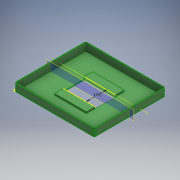
# Autodesk Inventor part: couvercle
Saved by Autodesk Inventor 2017 (Build 210142000, 142)
## iProperties
Part Number: couvercle
Material: Plastique ABS
Document SubType Name: Modeling
Designer: starl
Density: 1.06 g/cm^3
Appearance: Lisse - Blanc
Author: starl
Autodesk Inventor part; units mm, degrees
ref_plane "YZ Plane" through (0, 0, 0) normal (1, 0, 0) x (0, 1, 0)
ref_plane "XZ Plane" through (0, 0, 0) normal (0, 1, 0) x (-1, 0, 0)
ref_plane "XY Plane" through (0, 0, 0) normal (0, 0, 1) x (1, 0, 0)
sketch "Esquisse1" plane through (0, 0, 0) normal (0, 0, 1) x (1, 0, 0)
  line L0 (0, 0) -> (93, 0)
  line L1 (93, 0) -> (93, 83)
  line L2 (93, 83) -> (0, 83)
  line L3 (0, 83) -> (0, 0)
  line L4 (1, 1) -> (92, 1)
  line L5 (92, 1) -> (92, 82)
  line L6 (92, 82) -> (1, 82)
  line L7 (1, 82) -> (1, 1)
  dimension "d0" = 93
  dimension "d1" = 91
  dimension "d2" = 83
  dimension "d3" = 81
  dimension "d4" = 1
  dimension "d5" = 1
  constraints: 16 end point, 4 parallel, 2 horizontal, 2 perpendicular
  measures "d0" distance of L0.start L0.end
  measures "d1" distance of L4.start L4.end
  measures "d2" distance of L0.end L1.end
  measures "d3" distance of L4.end L5.end
  measures "d4" distance between parallel lines of L2 L6
  measures "d5" distance between parallel lines of L3 L7
extrude "Extrusion1" add sketch "Esquisse1" along normal blind 10 contours L3 L2 L1 L0 | L7 L6 L5 L4
shell "Coque1" thickness 1 removed faces 1 at (31, 55.3333, 10)
sketch "Esquisse2" plane through (1, 1, 1) normal (0, 0, 1) x (1, 0, 0)
  point P0 (-1, -1)
sketch "Esquisse3" plane through (1, 1, 1) normal (0, 0, 1) x (1, 0, 0)
  line L0 (63.2856, 52.5) -> (26.2856, 52.5)
  line L1 (26.2856, 52.5) -> (26.2856, 62.5)
  line L2 (26.2856, 62.5) -> (63.2856, 62.5)
  line L3 (63.2856, 62.5) -> (63.2856, 52.5)
  line L4 (0, 0) -> (91, 0) projected
  line L5 (91, 81) -> (0, 81) projected
  line L6 (0, 81) -> (0, 0) projected
  line L7 (92, -1) -> (92, 82) projected
  point P0 (-1, -1)
  point P1 (45.5, 0)
  point P2 (44.7856, 21.5)
  point P3 (44.7856, 52.5)
  point P4 (45.5, 81)
  point P5 (0, 40.5)
  point P6 (92, 40.5)
  point P7 (26.2856, 57.5)
  point P8 (-34.8368, 34.987)
  dimension "d11" = 37
  dimension "d12" = 10
  constraints: 8 end point, 6 midpoint, 2 parallel, 1 horizontal, 1 perpendicular
  measures "d11" distance of L0.start L0.end
  measures "d12" distance of L0.end L1.end
sketch "Esquisse4" plane through (1, 1, 1) normal (0, 0, 1) x (1, 0, 0)
  point P0 (-1, -1)
extrude "Extrusion3" add sketch "Esquisse3" along normal blind 2
shell "Coque3" thickness 0.2 removed faces 1 at (51.9523, 53.5, 1.6667)
ref_plane "Plan de construction1" through (1, 41.5, 1) normal (0, 1, 0) x (1, 0, 0)
mirror "Symétrie1" about plane through (1, 41.5, 1) normal (0, 1, 0) of "Extrusion3"
shell "Coque4" thickness 0.2 removed faces 1 at (51.9523, 29.5, 1.6667)
sketch "Esquisse5" plane through (1, 1, 3) normal (0, 0, 1) x (1, 0, 0)
  line L0 (26.2856, 52.5) -> (63.2856, 52.5) projected
  line L1 (26.2856, 28.5) -> (63.2856, 28.5) projected
  point P0 (-1, -1)
  dimension "d22" = 24
  measures "d22" distance between parallel lines of L0 L1
sketch "Esquisse6" plane through (0, 0, 0) normal (0, 0, -1) x (-1, 0, 0)
  line L0 (-64.2856, 53.5) -> (-28.2856, 53.5)
  line L1 (-28.2856, 53.5) -> (-28.2856, 29.5)
  line L2 (-28.2856, 29.5) -> (-64.2856, 29.5)
  line L3 (-64.2856, 29.5) -> (-64.2856, 53.5)
  line L4 (-64.0856, 53.5) -> (-27.4856, 53.5) projected
  line L5 (-64.2856, 29.5) -> (-64.2856, 19.5) projected
  point P0 (0, 0)
  dimension "d23" = 36
  dimension "d24" = 24
  constraints: 8 end point, 2 collinear, 2 parallel, 1 horizontal, 1 perpendicular
  measures "d23" distance of L0.start L0.end
  measures "d24" distance of L0.end L1.end
extrude "Extrusion4" cut sketch "Esquisse6" against normal blind 2
fillet "Congé1" radius 2 8 edges at (0, 83, 5) (46.5, 83, 0) (0, 41.5, 0) (93, 83, 5) (0, 0, 5) (93, 41.5, 0) (93, 0, 5) (46.5, 0, 0)
